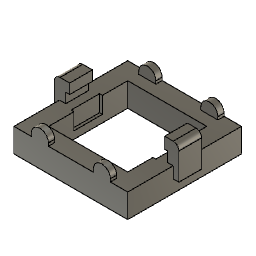
arc-board-mk2 v30 (Autodesk Fusion 360 archive; units mm, degrees)
design "mxledbit-switchbody"
part number: mxledbit container
Autodesk Fusion 360 part; units mm, degrees
sketch "Sketch1" plane through (0, 0, 0) normal (0, 0, 1) x (1, 0, 0) in component "main-switchbody"
  line L0 (0, 0) -> (0, 20) construction
  line L1 (0, 20) -> (20, 20) construction
  line L2 (20, 20) -> (20, 0) construction
  line L3 (20, 0) -> (0, 0) construction
  line L4 (0, 0) -> (20, 20) construction
  line L5 (20, 0) -> (0, 20) construction
  line L6 (10, 0) -> (18.9, 0) construction
  line L7 (10, 10) -> (18.9, 10) construction
  line L8 (18.9, 10) -> (18.9, 18.9) construction
  line L9 (18.9, 18.9) -> (1.1, 18.9) construction
  line L10 (1.1, 18.9) -> (1.1, 1.1) construction
  line L11 (1.1, 1.1) -> (18.9, 1.1) construction
  line L12 (18.9, 1.1) -> (18.9, 18.9) construction
  line L13 (10, 10) -> (3.05, 10) construction
  line L14 (3.05, 10) -> (3.05, 16.95) construction
  line L15 (3.05, 16.95) -> (16.95, 16.95) construction
  line L16 (16.95, 16.95) -> (16.95, 3.05) construction
  line L17 (16.95, 3.05) -> (3.05, 3.05) construction
  line L18 (3.05, 3.05) -> (3.05, 16.95) construction
  line L19 (3.05, 3.05) -> (0, 3.05) construction
  line L20 (3.05, 3.05) -> (3.05, 0) construction
  line L21 (16.95, 3.05) -> (20, 3.05) construction
  line L22 (16.95, 16.95) -> (20, 16.95) construction
  line L23 (16.95, 16.95) -> (16.95, 20) construction
  line L24 (3.05, 16.95) -> (3.05, 20) construction
  line L25 (3.05, 16.95) -> (0, 16.95) construction
  line L26 (3.05, 18.9) -> (6.05, 18.9) construction
  line L27 (6.05, 18.9) -> (6.05, 20) construction
  line L28 (16.95, 18.9) -> (13.95, 18.9) construction
  line L29 (13.95, 18.9) -> (13.95, 20) construction
  line L30 (16.95, 3.05) -> (16.95, 0) construction
  line L31 (16.95, 1.1) -> (13.95, 1.1) construction
  line L32 (13.95, 1.1) -> (13.95, 0) construction
  line L33 (3.05, 1.1) -> (6.05, 1.1) construction
  line L34 (6.05, 1.1) -> (6.05, 0) construction
  line L35 (0, 20) -> (20, 20) construction
  line L36 (20, 20) -> (20, 0) construction
  line L37 (20, 0) -> (0, 0) construction
  line L38 (0, 0) -> (0, 20) construction
  line L39 (0, 20) -> (20, 20)
  line L40 (20, 20) -> (20, 0)
  line L41 (20, 0) -> (0, 0)
  line L42 (0, 0) -> (0, 20)
  line L43 (16.95, 3.05) -> (3.05, 3.05)
  line L44 (3.05, 3.05) -> (3.05, 16.95)
  line L45 (3.05, 16.95) -> (16.95, 16.95)
  line L46 (16.95, 16.95) -> (16.95, 3.05)
  line L47 (3.05, 1.1) -> (6.05, 1.1)
  line L48 (6.05, 1.1) -> (6.05, 0)
  line L49 (6.05, 0) -> (3.05, 0)
  line L50 (3.05, 0) -> (3.05, 1.1)
  line L51 (13.95, 1.1) -> (16.95, 1.1)
  line L52 (16.95, 1.1) -> (16.95, 0)
  line L53 (16.95, 0) -> (13.95, 0)
  line L54 (13.95, 0) -> (13.95, 1.1)
  line L55 (13.95, 20) -> (16.95, 20)
  line L56 (16.95, 20) -> (16.95, 18.9)
  line L57 (16.95, 18.9) -> (13.95, 18.9)
  line L58 (13.95, 18.9) -> (13.95, 20)
  line L59 (3.05, 20) -> (6.05, 20)
  line L60 (6.05, 20) -> (6.05, 18.9)
  line L61 (6.05, 18.9) -> (3.05, 18.9)
  line L62 (3.05, 18.9) -> (3.05, 20)
  line L63 (1.1, 10) -> (1.1, 12)
  line L64 (1.1, 10) -> (1.1, 8)
  line L65 (1.1, 8) -> (-1.9, 8)
  line L66 (-1.9, 8) -> (1.1, 8)
  line L67 (1.1, 8) -> (1.1, 12)
  line L68 (1.1, 12) -> (-1.9, 12)
  line L69 (-1.9, 12) -> (-1.9, 8)
  line L70 (3.05, 10) -> (3.05, 7.5) construction
  line L71 (3.05, 7.5) -> (2.55, 7.5) construction
  line L72 (2.55, 7.5) -> (2.55, 12.5) construction
  line L73 (2.55, 12.5) -> (3.05, 12.5085) construction
  line L74 (3.05, 12.5085) -> (3.05, 7.5) construction
  line L75 (2.55, 12.5) -> (16.95, 12.5) construction
  line L76 (16.95, 12.5) -> (17.45, 12.5) construction
  line L77 (17.45, 12.5) -> (17.45, 7.5) construction
  line L78 (17.45, 7.5) -> (16.95, 7.5) construction
  line L79 (16.95, 7.5) -> (16.95, 12.5) construction
  line L80 (17.45, 7.5) -> (16.95, 7.5)
  line L81 (16.95, 7.5) -> (16.95, 12.5)
  line L82 (16.95, 12.5) -> (17.45, 12.5)
  line L83 (17.45, 12.5) -> (17.45, 7.5)
  line L84 (3.05, 7.5) -> (2.55, 7.5)
  line L85 (2.55, 7.5) -> (2.55, 12.5)
  line L86 (2.55, 12.5) -> (3.05, 12.5)
  line L87 (3.05, 12.5) -> (3.05, 7.5)
  dimension "d1" = 20
  dimension "d2" = 20
  dimension "d3" = 8.9
  dimension "d4" = 8.9
  dimension "d5" = 8.9
  dimension "d6" = 17.8
  dimension "d7" = 17.8
  dimension "d8" = 6.95
  dimension "d9" = 6.95
  dimension "d10" = 13.9
  dimension "d11" = 13.9
  dimension "d12" = 13.9
  dimension "d13" = 3
  dimension "d14" = 3
  dimension "d15" = 3
  dimension "d16" = 3
  dimension "d21" = 3
  dimension "d58" = 2.5
  dimension "d59" = 0.5
  dimension "d60" = 5
  dimension "d61" = 0.5
  dimension "d62" = 5
  constraint coincident L0.start L3.end
  constraint vertical L0
  constraint perpendicular L0 L1
  constraint perpendicular L1 L2
  constraint perpendicular L0 L3
  constraint midpoint L3 L6.start
  constraint parallel L3 L6
  constraint midpoint L4 L7.start
  constraint parallel L6 L7
  constraint perpendicular L7 L8
  constraint perpendicular L8 L9
  constraint perpendicular L9 L10
  constraint coincident L5 L11.end
  constraint perpendicular L10 L11
  constraint perpendicular L12 L13
  constraint perpendicular L13 L14
  constraint perpendicular L14 L15
  constraint perpendicular L7 L16
  constraint perpendicular L16 L17
  constraint coincident L0 L19.end
  constraint perpendicular L0 L19
  constraint coincident L3 L20.end
  constraint perpendicular L3 L20
  constraint coincident L2 L21.end
  constraint perpendicular L2 L21
  constraint coincident L2 L22.end
  constraint perpendicular L2 L22
  constraint coincident L1 L23.end
  constraint perpendicular L1 L23
  constraint coincident L1 L24.end
  constraint perpendicular L1 L24
  constraint coincident L0 L25.end
  constraint perpendicular L0 L25
  constraint coincident L24 L26.start
  constraint coincident L9 L26.start
  constraint coincident L9 L26.end
  constraint coincident L1 L27.end
  constraint perpendicular L1 L27
  constraint coincident L9 L28.start
  constraint coincident L23 L28.start
  constraint perpendicular L23 L28
  constraint coincident L1 L29.end
  constraint perpendicular L1 L29
  constraint coincident L6 L30.end
  constraint coincident L30 L31.start
  constraint coincident L11 L31.start
  constraint perpendicular L30 L31
  constraint coincident L6 L32.end
  constraint coincident L11 L33.start
  constraint coincident L20 L33.start
  constraint perpendicular L20 L33
  constraint coincident L3 L34.end
  constraint perpendicular L3 L34
  constraint horizontal L35
  constraint vertical L36
  constraint horizontal L37
  constraint vertical L38
  constraint horizontal L39
  constraint vertical L40
  constraint horizontal L41
  constraint vertical L42
  constraint horizontal L43
  constraint vertical L44
  constraint horizontal L45
  constraint vertical L46
  constraint horizontal L47
  constraint vertical L48
  constraint horizontal L49
  constraint vertical L50
  constraint horizontal L51
  constraint vertical L52
  constraint horizontal L53
  constraint vertical L54
  constraint horizontal L55
  constraint vertical L56
  constraint horizontal L57
  constraint vertical L58
  constraint horizontal L59
  constraint vertical L60
  constraint horizontal L61
  constraint vertical L62
  constraint midpoint L10 L63.start
  constraint coincident L10 L63.end
  constraint parallel L10 L63
  constraint coincident L10 L64.end
  constraint perpendicular L0 L65
  constraint horizontal L66
  constraint vertical L67
  constraint horizontal L68
  constraint vertical L69
  constraint perpendicular L13 L70
  constraint perpendicular L70 L71
  constraint perpendicular L71 L72
  constraint coincident L14 L73.end
  constraint perpendicular L71 L74
  constraint coincident L16 L75.end
  constraint perpendicular L16 L75
  constraint perpendicular L16 L76
  constraint perpendicular L76 L77
  constraint coincident L16 L78.end
  constraint perpendicular L16 L78
  constraint horizontal L80
  constraint vertical L81
  constraint horizontal L82
  constraint vertical L83
  constraint horizontal L84
  constraint vertical L85
  constraint horizontal L86
  constraint vertical L87
  measures "d1" distance of L0.start L0.end
  measures "d2" distance of L0.end L1.end
  measures "d3" distance of L6.start L6.end
  measures "d4" distance of L7.start L7.end
  measures "d5" distance of L7.end L8.end
  measures "d6" distance of L8.end L9.end
  measures "d7" distance of L9.end L10.end
  measures "d8" distance of L7.start L13.end
  measures "d9" distance of L13.end L14.end
  measures "d10" distance of L14.end L15.end
  measures "d11" distance of L15.end L16.end
  measures "d12" distance of L16.end L17.end
  measures "d13" distance of L26.start L26.end
  measures "d14" distance of L28.start L28.end
  measures "d15" distance of L31.start L31.end
  measures "d16" distance of L33.start L33.end
  measures "d21" distance of L64.end L65.end
  measures "d58" distance of L13.end L70.end
  measures "d59" distance of L70.end L71.end
  measures "d60" distance of L71.end L72.end
  measures "d61" distance of L75.end L76.end
  measures "d62" distance of L76.end L77.end
extrude "Extrude3" add sketch "Sketch1" along normal blind 7.5 contours L42 L63 L64 L65 L66 L67 L68 | L42 L65 L66 L68 L69 makes body 1 in component "main-switchbody"
extrude "Extrude2" add sketch "Sketch1" along normal blind 4 separate body contours L39 L40 L41 L42 L47 L48 L50 L51 L52 L54 L56 L57 L58 L60 L61 L62 L63 L64 L65 L66 L67 L68 | L42 L63 L64 L65 L66 L67 L68 | L46 L80 L81 L82 L83 | L44 L84 L85 L86 L87 makes body 2 in component "main-switchbody"
extrude "Extrude1" add sketch "Sketch1" along normal blind 6 separate body contours L39 L59 L60 L61 L62 | L39 L55 L56 L57 L58 | L41 L47 L48 L49 L50 | L41 L51 L52 L53 L54 makes body 3 at (4.05, 1.1, 2) makes body 4 at (5.05, 20, 4) makes body 5 at (14.95, 1.1, 2) makes body 6 at (14.95, 20, 2) in component "main-switchbody"
extrude "Extrude4" cut sketch "Sketch1" along normal blind 2 contours L42 L65 L66 L68 L69 bodies 1 in component "main-switchbody"
sketch "Sketch2" plane through (1.1, 0, 0) normal (1, 0, 0) x (0, 1, 0) in component "main-switchbody"
  line L0 (8, 0) -> (12, 0)
  line L1 (12, 0) -> (12, 7.5)
  line L2 (12, 7.5) -> (8, 7.5)
  line L3 (8, 7.5) -> (8, 0)
  line L4 (8, 7.5) -> (8, 4) construction
  line L5 (8, 4) -> (12, 4) construction
  line L6 (12, 4) -> (12, 7.5) construction
  line L7 (12, 7.5) -> (8, 7.5) construction
  line L8 (8, 7.5) -> (8, 5.75) construction
  line L9 (8, 5.75) -> (12, 5.75) construction
  line L10 (8, 7.5) -> (12, 7.5)
  line L11 (12, 7.5) -> (12, 5.75)
  line L12 (12, 5.75) -> (8, 5.75)
  line L13 (8, 5.75) -> (8, 7.5)
  dimension "d26" = 1.75
  constraint coincident L2.end L3.start
  constraint coincident L3 L4.end
  constraint perpendicular L2 L4
  constraint coincident L1 L5.end
  constraint perpendicular L1 L5
  constraint coincident L1.end L2.start
  constraint perpendicular L2 L6
  constraint perpendicular L5 L8
  constraint midpoint L6 L9.end
  constraint horizontal L10
  constraint vertical L11
  constraint horizontal L12
  constraint vertical L13
  measures "d26" distance of L2.end L8.end
extrude "Extrude5" add sketch "Sketch2" along normal blind 1 contours L1 L2 L3 L10 L11 L12 L13 bodies 1 in component "main-switchbody"
extrude "Extrude6" cut 1 faces at (-1.9, 10.6667, 3.8333) along direction (1, 0, 0) blind 1 on bodies 1 bodies 1 in component "main-switchbody"
sketch "Sketch3" plane through (0, 18.9, 0) normal (0, -1, 0) x (1, 0, 0) in component "main-switchbody"
  line L0 (3.05, 0) -> (6.05, 0)
  line L1 (6.05, 0) -> (6.05, 6)
  line L2 (6.05, 6) -> (3.05, 6)
  line L3 (3.05, 6) -> (3.05, 0)
  line L4 (3.05, 6) -> (3.05, 4) construction
  line L5 (6.05, 4) -> (6.05, 6) construction
  line L6 (3.05, 6) -> (3.05, 4.5) construction
  line L7 (6.05, 6) -> (6.05, 4.5) construction
  arc A0 (6.05, 4.5) -> (3.05, 4.5) centre (4.55, 4.5) ccw construction
  arc A1 (6.05, 4.5) -> (3.05, 4.5) centre (4.55, 4.5) ccw
  dimension "d31" = 1.5
  dimension "d32" = 1.5
  constraint coincident L2.end L3.start
  constraint coincident L3 L4.end
  constraint perpendicular L2 L4
  constraint coincident L1 L5.start
  constraint coincident L1.end L2.start
  constraint perpendicular L2 L5
  constraint perpendicular L2 L6
  constraint perpendicular L2 L7
  constraint tangent L2 A0
  constraint tangent L2 A1
  measures "d31" distance of L2.end L6.end
  measures "d32" distance of L1.end L7.end
extrude "Extrude7" cut sketch "Sketch3" against normal blind 1.1 contours L2 L3 A1 | L1 L2 A1 bodies 4 in component "main-switchbody"
sketch "Sketch4" plane through (0, 0, 0) normal (0, -1, 0) x (1, 0, 0) in component "main-switchbody"
  line L0 (3.05, 0) -> (6.05, 0)
  line L1 (6.05, 0) -> (6.05, 6)
  line L2 (6.05, 6) -> (3.05, 6)
  line L3 (3.05, 6) -> (3.05, 0)
  line L4 (3.05, 6) -> (3.05, 4.5) construction
  line L5 (6.05, 6) -> (6.05, 4.5) construction
  arc A0 (6.05, 4.5) -> (3.05, 4.5) centre (4.55, 4.5) ccw
  constraint coincident L2.end L3.start
  constraint coincident L3 L4.end
  constraint perpendicular L2 L4
  constraint coincident L1.end L2.start
  constraint coincident L1 L5.end
  constraint perpendicular L2 L5
  constraint tangent L2 A0
extrude "Extrude8" cut sketch "Sketch4" against normal blind 1.1 contours L2 L3 A0 | L1 L2 A0 bodies 3 in component "main-switchbody"
sketch "Sketch5" plane through (0, 0, 0) normal (0, -1, 0) x (1, 0, 0) in component "main-switchbody"
  line L0 (13.95, 0) -> (16.95, 0)
  line L1 (16.95, 0) -> (16.95, 6)
  line L2 (16.95, 6) -> (13.95, 6)
  line L3 (13.95, 6) -> (13.95, 0)
  line L4 (13.95, 6) -> (13.95, 4.5) construction
  line L5 (16.95, 6) -> (16.95, 4.5) construction
  arc A0 (16.95, 4.5) -> (13.95, 4.5) centre (15.45, 4.5) ccw
  constraint coincident L2.end L3.start
  constraint coincident L3 L4.end
  constraint perpendicular L2 L4
  constraint coincident L1.end L2.start
  constraint coincident L1 L5.end
  constraint perpendicular L2 L5
  constraint tangent L2 A0
extrude "Extrude9" cut sketch "Sketch5" against normal blind 1.1 contours L2 L3 A0 | L1 L2 A0 bodies 5 in component "main-switchbody"
sketch "Sketch6" plane through (0, 18.9, 0) normal (0, -1, 0) x (1, 0, 0) in component "main-switchbody"
  line L0 (13.95, 0) -> (16.95, 0)
  line L1 (16.95, 0) -> (16.95, 6)
  line L2 (16.95, 6) -> (13.95, 6)
  line L3 (13.95, 6) -> (13.95, 0)
  line L4 (13.95, 6) -> (13.95, 4.5) construction
  line L5 (16.95, 6) -> (16.95, 4.5) construction
  arc A0 (16.95, 4.5) -> (13.95, 4.5) centre (15.45, 4.5) ccw
  constraint coincident L2.end L3.start
  constraint coincident L3 L4.end
  constraint perpendicular L2 L4
  constraint coincident L1.end L2.start
  constraint coincident L1 L5.end
  constraint perpendicular L2 L5
  constraint tangent L2 A0
extrude "Extrude10" cut sketch "Sketch6" against normal blind 1.1 contours L2 L3 A0 | L1 L2 A0 bodies 6 in component "main-switchbody"
sketch "Sketch7" plane through (0, 0, 4) normal (0, 0, 1) x (-1, 0, 0) in component "main-switchbody"
  line L0 (-3.05, -16.95) -> (-16.95, -16.95)
  line L1 (-16.95, -16.95) -> (-16.95, -3.05)
  line L2 (-16.95, -3.05) -> (-3.05, -3.05)
  line L3 (-3.05, -3.05) -> (-3.05, -16.95)
  line L4 (-6.05, -20) -> (-6.05, -18.9)
  line L5 (-6.05, -18.9) -> (-3.05, -18.9)
  line L6 (-3.05, -18.9) -> (-3.05, -20)
  line L7 (-3.05, -20) -> (0, -20)
  line L8 (0, -20) -> (0, 0)
  line L9 (0, 0) -> (-3.05, 0)
  line L10 (-3.05, 0) -> (-3.05, -1.1)
  line L11 (-3.05, -1.1) -> (-6.05, -1.1)
  line L12 (-6.05, -1.1) -> (-6.05, 0)
  line L13 (-6.05, 0) -> (-13.95, 0)
  line L14 (-13.95, 0) -> (-13.95, -1.1)
  line L15 (-13.95, -1.1) -> (-16.95, -1.1)
  line L16 (-16.95, -1.1) -> (-16.95, 0)
  line L17 (-16.95, 0) -> (-20, 0)
  line L18 (-20, 0) -> (-20, -20)
  line L19 (-20, -20) -> (-16.95, -20)
  line L20 (-16.95, -20) -> (-16.95, -18.9)
  line L21 (-16.95, -18.9) -> (-13.95, -18.9)
  line L22 (-13.95, -18.9) -> (-13.95, -20)
  line L23 (-13.95, -20) -> (-6.05, -20)
  line L24 (-20, -10) -> (-20, -11.5) construction
  line L25 (-20, -10) -> (-20, -8.5) construction
  line L26 (-20, -8.5) -> (-19, -8.5) construction
  line L27 (-19, -8.5) -> (-19, -11.5) construction
  line L28 (-19, -11.5) -> (-20, -11.5) construction
  line L29 (-20, -11.5) -> (-21, -11.5) construction
  line L30 (-21, -11.5) -> (-21, -8.5) construction
  line L31 (-21, -8.5) -> (-20, -8.5) construction
  line L32 (-19, -11.5) -> (-21, -11.5)
  line L33 (-21, -11.5) -> (-21, -8.5)
  line L34 (-21, -8.5) -> (-19, -8.5)
  line L35 (-19, -8.5) -> (-19, -11.5)
  dimension "d41" = 1.5
  dimension "d42" = 1
  constraint midpoint L18 L24.start
  constraint parallel L18 L24
  constraint coincident L18 L25.end
  constraint parallel L18 L25
  constraint perpendicular L25 L26
  constraint perpendicular L26 L27
  constraint perpendicular L24 L29
  constraint perpendicular L29 L30
  constraint horizontal L32
  constraint vertical L33
  constraint horizontal L34
  constraint vertical L35
  measures "d41" distance of L24.start L24.end
  measures "d42" distance of L24.end L29.end
extrude "Extrude11" add sketch "Sketch7" along normal blind 3 contours L18 L32 L33 L34 | L18 L32 L34 L35 bodies 2 in component "main-switchbody"
extrude "Extrude12" add 1 faces at (20, 8.5, 6) along direction (0, -1, 0) blind 0.5 on bodies 2 bodies 2 in component "main-switchbody"
extrude "Extrude13" add 1 faces at (20, 11.5, 6) along direction (0, 1, 0) blind 0.5 on bodies 2 bodies 2 in component "main-switchbody"
extrude "Extrude14" add 1 faces at (20.3333, 10.6667, 7) along direction (0, 0, 1) blind 0.75 on bodies 2 bodies 2 in component "main-switchbody"
sketch "Sketch8" plane through (0, 0, 4) normal (0, 0, -1) x (1, 0, 0) in component "main-switchbody"
  line L0 (20, -8) -> (20, -12)
  line L1 (20, -12) -> (21, -12)
  line L2 (21, -12) -> (21, -8)
  line L3 (21, -8) -> (20, -8)
  line L4 (20, -12) -> (20, -8)
  constraint coincident L0.end L1.start
  constraint coincident L0.start L3.end
extrude "Extrude15" add sketch "Sketch8" along normal blind 2 bodies 2 in component "main-switchbody"
sketch "Sketch9" plane through (19, 0, 0) normal (-1, 0, 0) x (0, -1, 0) in component "main-switchbody"
  line L0 (-12, 4) -> (-8, 4)
  line L1 (-8, 4) -> (-8, 7.75)
  line L2 (-8, 7.75) -> (-12, 7.75)
  line L3 (-12, 7.75) -> (-12, 4)
  line L4 (-12, 7.75) -> (-12, 5.75) construction
  line L5 (-12, 5.75) -> (-8, 5.75) construction
  line L6 (-12, 7.75) -> (-8, 7.75)
  line L7 (-8, 7.75) -> (-8, 5.75)
  line L8 (-8, 5.75) -> (-12, 5.75)
  line L9 (-12, 5.75) -> (-12, 7.75)
  dimension "d53" = 2
  constraint coincident L2.end L3.start
  constraint perpendicular L2 L4
  constraint coincident L1 L5.end
  constraint perpendicular L1 L5
  constraint horizontal L6
  constraint vertical L7
  constraint horizontal L8
  constraint vertical L9
  measures "d53" distance of L2.end L4.end
extrude "Extrude16" add sketch "Sketch9" along normal blind 0.5 contours L1 L2 L3 L6 L7 L8 L9 bodies 2 in component "main-switchbody"
extrude "Extrude17" cut 1 faces at (2.1, 9.3333, 6.9167) along direction (-1, 0, 0) blind 0.3 on bodies 1 bodies 1 in component "main-switchbody"
extrude "Extrude18" cut sketch "Sketch1" along normal blind 2.7 contours L44 L84 L85 L86 L87 bodies 2 in component "main-switchbody"
extrude "Extrude19" cut sketch "Sketch1" along normal blind 2.7 contours L46 L80 L81 L82 L83 bodies 2 in component "main-switchbody"
extrude "Extrude20" add sketch "Sketch1" against normal blind 0.2 contours L39 L40 L41 L42 L47 L48 L50 L51 L52 L54 L56 L57 L58 L60 L61 L62 L63 L64 L65 L66 L67 L68 | L39 L59 L60 L61 L62 | L42 L63 L64 L65 L66 L67 L68 | L39 L55 L56 L57 L58 | L41 L47 L48 L49 L50 | L41 L51 L52 L53 L54 bodies 1 2 3 4 5 6 in component "main-switchbody"
fillet "Fillet1" radius 1 2 edges at (21, 10, 7.75) (-0.9, 10, 7.5) on bodies 1 in component "main-switchbody"
extrude "Extrude21" add 1 faces at (2.8833, 9.1667, 2.7) along direction (0, 0, -1) blind 2.9 on bodies 1 bodies 1 in component "main-switchbody"
extrude "Extrude22" add 1 faces at (17.1167, 10.8333, 2.7) along direction (0, 0, -1) blind 2.9 on bodies 1 bodies 1 in component "main-switchbody"
sketch "Sketch10" plane through (0, 0, 4) normal (0, 0, 1) x (-1, 0, 0) in component "main-switchbody"
  line L0 (-3.05, -16.95) -> (-16.95, -16.95)
  line L1 (-16.95, -16.95) -> (-16.95, -3.05)
  line L2 (-16.95, -3.05) -> (-3.05, -3.05)
  line L3 (-3.05, -3.05) -> (-3.05, -16.95)
  line L4 (0, -12) -> (-1.1, -12)
  line L5 (-1.1, -12) -> (-1.1, -8)
  line L6 (-1.1, -8) -> (0, -8)
  line L7 (0, -8) -> (0, 0)
  line L8 (0, 0) -> (-3.05, 0)
  line L9 (-3.05, 0) -> (-3.05, -1.1)
  line L10 (-3.05, -1.1) -> (-6.05, -1.1)
  line L11 (-6.05, -1.1) -> (-6.05, 0)
  line L12 (-6.05, 0) -> (-13.95, 0)
  line L13 (-13.95, 0) -> (-13.95, -1.1)
  line L14 (-13.95, -1.1) -> (-16.95, -1.1)
  line L15 (-16.95, -1.1) -> (-16.95, 0)
  line L16 (-16.95, 0) -> (-20, 0)
  line L17 (-20, 0) -> (-20, -8)
  line L18 (-20, -8) -> (-19, -8)
  line L19 (-19, -8) -> (-19, -12)
  line L20 (-19, -12) -> (-20, -12)
  line L21 (-20, -12) -> (-20, -20)
  line L22 (-20, -20) -> (-16.95, -20)
  line L23 (-16.95, -20) -> (-16.95, -18.9)
  line L24 (-16.95, -18.9) -> (-13.95, -18.9)
  line L25 (-13.95, -18.9) -> (-13.95, -20)
  line L26 (-13.95, -20) -> (-6.05, -20)
  line L27 (-6.05, -20) -> (-6.05, -18.9)
  line L28 (-6.05, -18.9) -> (-3.05, -18.9)
  line L29 (-3.05, -18.9) -> (-3.05, -20)
  line L30 (-3.05, -20) -> (0, -20)
  line L31 (0, -20) -> (0, -12)
  line L32 (-3.05, -10) -> (-3.05, -12.5) construction
  line L33 (-3.05, -12.5) -> (-3.05, -7.5) construction
  line L34 (-3.05, -7.5) -> (-2.55, -7.5) construction
  line L35 (-2.55, -7.5) -> (-3.05, -7.5) construction
  line L36 (-3.05, -7.5) -> (-3.05, -12.5) construction
  line L37 (-3.05, -12.5) -> (-2.55, -12.5) construction
  line L38 (-2.55, -12.5) -> (-2.55, -7.5) construction
  line L39 (-3.05, -12.5) -> (-16.95, -12.5) construction
  line L40 (-16.95, -12.5) -> (-16.95, -7.5) construction
  line L41 (-16.95, -7.5) -> (-17.45, -7.5) construction
  line L42 (-17.45, -7.5) -> (-16.95, -7.5) construction
  line L43 (-16.95, -7.5) -> (-16.95, -12.5) construction
  line L44 (-16.95, -12.5) -> (-17.45, -12.5) construction
  line L45 (-17.45, -12.5) -> (-17.45, -7.5) construction
  line L46 (-16.95, -12.5) -> (-17.45, -12.5)
  line L47 (-17.45, -12.5) -> (-17.45, -7.5)
  line L48 (-17.45, -7.5) -> (-16.95, -7.5)
  line L49 (-16.95, -7.5) -> (-16.95, -12.5)
  line L50 (-2.55, -12.5) -> (-3.05, -12.5)
  line L51 (-3.05, -12.5) -> (-3.05, -7.5)
  line L52 (-3.05, -7.5) -> (-2.55, -7.5)
  line L53 (-2.55, -7.5) -> (-2.55, -12.5)
  dimension "d75" = 5
  dimension "d76" = 0.5
  dimension "d77" = 0.5
  constraint midpoint L3 L32.start
  constraint coincident L3 L32.end
  constraint perpendicular L0 L32
  constraint parallel L3 L33
  constraint perpendicular L33 L34
  constraint horizontal L35
  constraint vertical L36
  constraint horizontal L37
  constraint vertical L38
  constraint coincident L1 L39.end
  constraint perpendicular L1 L39
  constraint coincident L1 L40.end
  constraint perpendicular L39 L40
  constraint perpendicular L40 L41
  constraint horizontal L42
  constraint vertical L43
  constraint horizontal L44
  constraint vertical L45
  constraint horizontal L46
  constraint vertical L47
  constraint horizontal L48
  constraint vertical L49
  constraint horizontal L50
  constraint vertical L51
  constraint horizontal L52
  constraint vertical L53
  measures "d75" distance of L32.end L33.end
  measures "d76" distance of L33.end L34.end
  measures "d77" distance of L40.end L41.end
extrude "Extrude23" cut sketch "Sketch10" against normal blind 2.9 contours L3 L50 L51 L52 L53 | L1 L46 L47 L48 L49 bodies 1 in component "main-switchbody"
component "main-switchbody" placed x (1, 0, 0) y (0, 1, 0) z (0, 0, 1) at (1.4919, -0.7126, 1.0152)
